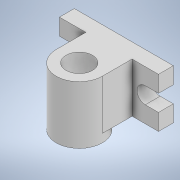
# Autodesk Inventor part: 2-5
Saved by Autodesk Inventor 2020 (Build 240168000, 168)
## iProperties
Created: 2023-12-07
Part Number: 2-5
Material: 常规
Document SubType Name: Modeling
Designer: Z
Density: 1 g/cm^3
Appearance: 默认
Author: Z
Autodesk Inventor part; units mm, degrees
ref_plane "YZ Plane" through (0, 0, 0) normal (1, 0, 0) x (0, 1, 0)
ref_plane "XZ Plane" through (0, 0, 0) normal (0, 1, 0) x (-1, 0, 0)
ref_plane "XY Plane" through (0, 0, 0) normal (0, 0, 1) x (1, 0, 0)
sketch "草图1" plane through (0, 0, 0) normal (0, 0, 1) x (1, 0, 0)
  line L0 (-30, 15) -> (30, 15)
  line L1 (30, -15) -> (-30, -15)
  line L2 (-30, 15) -> (30, -15) construction
  line L3 (30, 15) -> (-30, -15) construction
  arc A0 (-22, -5) -> (-22, 5) centre (-22, 0) ccw
  line L4 (-22, 5) -> (-30, 5)
  line L5 (-22, -5) -> (-30, -5)
  line L6 (-30, -15) -> (-30, -5)
  line L7 (-30, 5) -> (-30, 15)
  arc A1 (22, 5) -> (22, -5) centre (22, 0) ccw
  line L8 (22, 5) -> (30, 5)
  line L9 (22, -5) -> (30, -5)
  line L10 (30, 15) -> (30, 5)
  line L11 (30, -5) -> (30, -15)
  point P0 (0, 0)
  dimension "d0" = 60
  dimension "d1" = 30
  dimension "d3" = 10
  dimension "d5" = 10
  constraints: 24 end point, 10 perpendicular, 5 parallel, 4 point on circle, 3 tangent, 2 centre point, 2 midpoint, 1 horizontal
  measures "d0" distance of L1.start L1.end
  measures "d1" distance of L0.end L1.start
  measures "d3" diameter of A0
  measures "d5" diameter of A1
extrude "拉伸1" add sketch "草图1" along normal blind 9
sketch "草图2" plane through (-30, -15, 0) normal (0, -1, 0) x (1, 0, 0)
  line L0 (30, 0) -> (30, 27)
  circle A0 centre (30, 27) radius 8
  circle A1 centre (30, 27) radius 14
  line L1 (60, 9) -> (0, 9) projected
  line L2 (44, 27) -> (44, 9)
  line L3 (16, 27) -> (16, 9)
  dimension "d8" = 27
  dimension "d9" = 16
  dimension "d10" = 28
  constraints: 6 end point, 2 centre point, 2 coincident, 2 perpendicular, 2 point on circle, 2 point on line, 2 tangent, 1 vertical
  measures "d8" distance of L0.start L0.end
  measures "d9" diameter of A0
  measures "d10" diameter of A1
extrude "拉伸2" add sketch "草图2" against normal blind 30
sketch "草图3" plane through (-30, -15, 0) normal (0, -1, 0) x (1, 0, 0)
  line L0 (30, 0) -> (30, 27)
  circle A0 centre (30, 27) radius 14
  circle A1 centre (30, 27) radius 8
  dimension "d13" = 27
  dimension "d14" = 28
  dimension "d15" = 16
  constraints: 2 centre point, 2 coincident, 2 end point, 1 vertical
  measures "d13" distance of L0.start L0.end
  measures "d14" diameter of A0
  measures "d15" diameter of A1
extrude "拉伸3" add sketch "草图3" along normal blind 5
